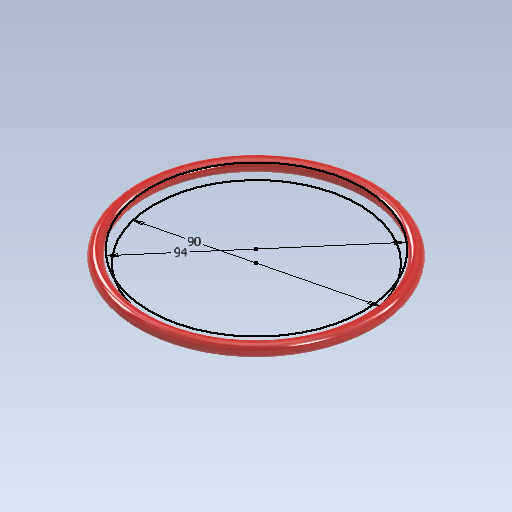
# Autodesk Inventor part: Sello Plato Oring 2-343
Saved by Autodesk Inventor 2020 (Build 240168000, 168)
## iProperties
Created: 2020-06-24
Part Number: Sello Plato Oring 2-343
Material: Rubber, Silicone
Document SubType Name: Modeling
Designer: Juan
Density: 1.25 g/cm^3
Appearance: Orange-Red
Author: Juan
Autodesk Inventor part; units mm, degrees
ref_plane "YZ Plane" through (0, 0, 0) normal (1, 0, 0) x (0, 1, 0)
ref_plane "XY Plane" through (0, 0, 0) normal (0, 0, 1) x (1, 0, 0)
sketch "Sketch1" plane through (0, 0, 0) normal (1, 0, 0) x (0, 1, 0)
  circle A0 centre (0, 49.975) radius 2.665
  line L0 (0, 0) -> (2.0054, 0)
  dimension "d0" = 5.33
  dimension "d1" = 49.975
  constraints: 2 end point, 1 centre point, 1 horizontal
  measures "d0" diameter of A0
  measures "d1" distance of L0.start A0.centre
revolve "Revolution1" add sketch "Sketch1" angle 360 about axis through (0, 0, 0) along (0, 1, 0)
ref_plane "Work Plane2" through (0, -2.665, 0) normal (0, 1, 0) x (-1, 0, 0)
ref_plane "Work Plane1" through (0, 2.665, 0) normal (0, 1, 0) x (-1, 0, 0)
sketch "Sketch2" plane through (0, 2.665, 0) normal (0, 1, 0) x (-1, 0, 0)
  circle A0 centre (0, 0) radius 47
  dimension "d5" = 94
  constraints: 1 centre point, 1 coincident
  measures "d5" diameter of A0
sketch "Sketch3" plane through (0, -2.665, 0) normal (0, 1, 0) x (-1, 0, 0)
  circle A0 centre (0, 0) radius 45
  dimension "d6" = 90
  constraints: 1 centre point, 1 coincident
  measures "d6" diameter of A0
body "Solid1"
